bagues_fusion_parametrique (Autodesk Fusion 360 design; units mm, degrees)
part number: 2026-05-13-14-20-41-796
Autodesk Fusion 360 part; units mm, degrees
sketch "Esquisse8" plane through (0, 0, 0) normal (0, 1, 0) x (1, 0, 0)
  line L0 (50, 0) -> (61, 0)
  line L1 (61, 0) -> (61, 10)
  line L2 (61, 10) -> (65, 10)
  line L3 (65, 10) -> (65, 0)
  line L4 (65, 0) -> (69, 0)
  line L5 (69, 0) -> (69, 50)
  line L6 (69, 50) -> (55, 50)
  line L7 (55, 50) -> (55, 25)
  line L8 (55, 25) -> (50, 25)
  line L9 (50, 25) -> (50, 0)
revolve "Révolution7" add sketch "Esquisse8" angle 360 about axis through (0, 0, 1.75) along (0, 0, 1) makes body 1
sketch "Esquisse9" plane through (0, 0, 0) normal (0, 1, 0) x (1, 0, 0)
  line L0 (50, 0) -> (61, 0)
  line L1 (61, 0) -> (61, 10)
  line L2 (61, 10) -> (65, 10)
  line L3 (65, 10) -> (65, 0)
  line L4 (65, 0) -> (69, 0)
  line L5 (69, 0) -> (69, 50)
  line L6 (69, 50) -> (55, 50)
  line L7 (55, 50) -> (55, 75)
  line L8 (55, 75) -> (50, 75)
  line L9 (50, 75) -> (50, 0)
revolve "Révolution8" add sketch "Esquisse9" angle 360 about axis through (0, 0, 1.75) along (0, 0, 1) separate body makes body 2
move_body "Déplacer6" bodies 2 to x (1, 0, 0) y (0, 1, 0) z (0, 0, 1) at (158, 0, 0)
thread "Filetage7" "ISO Metric profile 110.0 M110x6 M110x6 6H" major diameter 110.633 minor diameter 103.9048 pitch 6 angle 60 modelled right hand crest width 1.6155 on face at (54.9316, -2.7415, -41.6667) crest through (51.9524, 0, -48.5) on bodies 1
thread "Filetage8" "ISO Metric profile 110.0 M110x6 M110x6 6g" major diameter 109.62 minor diameter 102.7258 pitch 6 angle 60 modelled right hand crest width 0.8366 on face at (212.9316, -2.7415, -58.3333) crest through (212.81, 0, -76.5) on bodies 2
named bodies: "Bague_Femelle", "Bague_Male"
